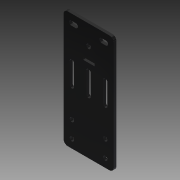
# Autodesk Inventor part: S2_ep
Saved by Autodesk Inventor 2014 (Build 180170000, 170)
## iProperties
Category: Open hardware
Company: www.shapeoko.com
Created: 2013-02-18
Part Number: S2_ep
Material: Steel, Mild
Document SubType Name: Modeling
Designer: Edward
Density: 1 g/cm^3
Project: Shapeoko v2.0
Catalog Web Link: www.shapeoko.com
Description: End Plate
Stock Number: S2_ep
Vendor: tdolan
Appearance: Lacquer - Black
Author: Edward
Title: End Plates
Subject: Shapeoko v2.0
Revision Number: 1
Autodesk Inventor part; units mm, degrees
ref_plane "YZ Plane" through (0, 0, 0) normal (1, 0, 0) x (0, 1, 0)
ref_plane "XZ Plane" through (0, 0, 0) normal (0, 1, 0) x (-1, 0, 0)
ref_plane "XY Plane" through (0, 0, 0) normal (0, 0, 1) x (1, 0, 0)
sketch "Sketch1" plane through (0, 0, 0) normal (0, 0, 1) x (1, 0, 0)
  line L0 (-30, 70) -> (30, 70)
  line L1 (30, 70) -> (30, -70)
  line L2 (30, -70) -> (-30, -70)
  line L3 (-30, -70) -> (-30, 70)
  point P0 (0, 0)
  dimension "d0" = 60
  dimension "d1" = 140
  dimension "d2" = 30
  dimension "d3" = 70
  constraints: 8 end point, 2 parallel, 1 horizontal, 1 perpendicular
  measures "d0" distance of L1.end L2.end
  measures "d1" distance of L0.end L1.end
  measures "d2" distance from line of point (0, 0) L3
  measures "d3" distance from line of L0 point (0, 0)
extrude "Extrusion1" add sketch "Sketch1" along normal blind 3.4163
sketch "Sketch2" plane through (0, 0, 3.4163) normal (0, 0, 1) x (1, 0, 0)
  line L0 (-30, 70) -> (-30, -70) projected
  line L1 (-30, -70) -> (30, -70) projected
  circle A0 centre (-20, -60) radius 2.625
  point P0 (0, 0)
  dimension "d6" = 5.25
  dimension "d7" = 10
  dimension "d8" = 10
  constraints: 1 centre point
  measures "d6" diameter of A0
  measures "d7" distance from line of L1 A0.centre
  measures "d8" distance from line of L0 A0.centre
extrude "Extrusion2" cut sketch "Sketch2" against normal through all
pattern_linear "Rectangular Pattern1" count 2 spacing 40 along (1, 0, 0) count 2 spacing 20 along (0, 1, 0) of "Extrusion2"
sketch "Sketch3" plane through (0, 0, 3.4163) normal (0, 0, 1) x (1, 0, 0)
  line L0 (-30, 70) -> (-30, -70) projected
  line L1 (-30, -70) -> (30, -70) projected
  arc A0 (-22.625, -5) -> (-17.375, -5) centre (-20, -5) ccw
  arc A1 (-17.375, 20) -> (-22.625, 20) centre (-20, 20) ccw
  line L2 (-22.625, 20) -> (-22.625, -5)
  line L3 (-17.375, -5) -> (-17.375, 20)
  point P0 (0, 0)
  dimension "d17" = 5.25
  dimension "d18" = 65
  dimension "d19" = 10
  dimension "d20" = 5.25
  dimension "d22" = 10
  dimension "d26" = 25
  dimension "d27" = 25
  constraints: 4 end point, 4 point on circle, 3 tangent, 2 centre point
  measures "d17" diameter of A0
  measures "d18" distance from line of L1 A0.centre
  measures "d19" distance from line of L0 A0.centre
  measures "d20" diameter of A1
  measures "d22" distance from line of L0 A1.centre
  measures "d26" distance of A0.centre A1.centre
  measures "d27" distance of L3.start L3.end
extrude "Extrusion3" cut sketch "Sketch3" against normal through all
sketch "Sketch4" plane through (0, 0, 3.4163) normal (0, 0, 1) x (1, 0, 0)
  line L0 (-30, 70) -> (-30, -70) projected
  line L1 (-30, -70) -> (30, -70) projected
  line L2 (-6.5, 32) -> (7.5, 32)
  line L3 (7.5, 32) -> (7.5, 29)
  line L4 (7.5, 29) -> (-6.5, 29)
  line L5 (-6.5, 29) -> (-6.5, 32)
  point P0 (0, 0)
  dimension "d28" = 14
  dimension "d29" = 3
  dimension "d30" = 99
  dimension "d31" = 23.5
  constraints: 8 end point, 2 parallel, 1 horizontal, 1 perpendicular
  measures "d28" distance of L3.end L4.end
  measures "d29" distance of L2.end L3.end
  measures "d30" distance between parallel lines of L1 L4
  measures "d31" distance between parallel lines of L0 L5
extrude "Extrusion4" cut sketch "Sketch4" against normal through all
sketch "Sketch5" plane through (0, 0, 3.4163) normal (0, 0, 1) x (1, 0, 0)
  line L0 (30, 70) -> (-30, 70) projected
  line L1 (-30, 70) -> (-30, -70) projected
  line L2 (-30, -70) -> (30, -70) projected
  circle A0 centre (0, 46) radius 2.625
  arc A1 (-20.625, 62.625) -> (-20.625, 57.375) centre (-20.625, 60) ccw
  arc A2 (15.625, 62.625) -> (15.625, 57.375) centre (15.625, 60) ccw
  arc A3 (-15.375, 57.375) -> (-15.375, 62.625) centre (-15.375, 60) ccw
  line L3 (-20.625, 62.625) -> (-15.375, 62.625)
  line L4 (-15.375, 57.375) -> (-20.625, 57.375)
  arc A4 (20.875, 57.375) -> (20.875, 62.625) centre (20.875, 60) ccw
  line L5 (20.875, 62.625) -> (15.625, 62.625)
  line L6 (15.625, 57.375) -> (20.875, 57.375)
  point P0 (0, 0)
  dimension "d34" = 5.25
  dimension "d35" = 116
  dimension "d36" = 5.25
  dimension "d37" = 5.25
  dimension "d38" = 10
  dimension "d39" = 10
  dimension "d40" = 36.25
  dimension "d41" = 9.375
  dimension "d48" = 5.25
  dimension "d49" = 5.25
  dimension "d50" = 10
  dimension "d51" = 5.25
  dimension "d52" = 5.25
  dimension "d53" = 5.25
  dimension "d54" = 10
  dimension "d55" = 5.25
  constraints: 8 end point, 8 point on circle, 6 tangent, 5 centre point
  measures "d34" diameter of A0
  measures "d35" distance from line of L2 A0.centre
  measures "d36" diameter of A1
  measures "d37" diameter of A2
  measures "d38" distance from line of L0 A1.centre
  measures "d39" distance from line of L0 A2.centre
  measures "d40" distance of A1.centre A2.centre
  measures "d41" distance from line of L1 A1.centre
  measures "d48" diameter of A3
  measures "d49" distance of A1.centre A3.centre
  measures "d50" distance from line of L0 A3.centre
  measures "d51" distance of L3.start L3.end
  measures "d52" diameter of A4
  measures "d53" distance of A2.centre A4.centre
  measures "d54" distance from line of L0 A4.centre
  measures "d55" distance of L6.start L6.end
extrude "Extrusion5" cut sketch "Sketch5" against normal blind 3.4163
pattern_linear "Rectangular Pattern2" count 3 spacing 20 along (1, 0, 0) of "Extrusion3"
fillet "Fillet1" radius 5 4 edges at (-30, 70, 1.7082) (30, 70, 1.7082) (30, -70, 1.7082) (-30, -70, 1.7082)
equation "\"d2\" = 0.5 * d0"
equation "\"d3\" = 0.5 * d1"
equation "\"d20\" = d17"
equation "\"d39\" = d38"
body "Solid1"
